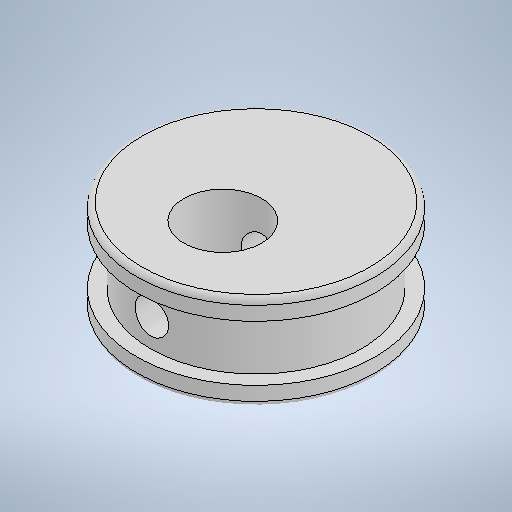
# Autodesk Inventor part: 204
Saved by Autodesk Inventor 2025 (Build 290162010, 162A)
## iProperties
Created: 2024-05-30
Part Number: 204
Material: Generic
Document SubType Name: Modeling
Designer: Fabri
Density: 1 g/cm^3
Appearance: Default
Author: Fabri
Autodesk Inventor part; units mm, degrees
ref_plane "YZ Plane" through (0, 0, 0) normal (1, 0, 0) x (0, 1, 0)
ref_plane "XY Plane" through (0, 0, 0) normal (0, 0, 1) x (1, 0, 0)
sketch "Sketch1" plane through (0, 0, 0) normal (0, 1, 0) x (-1, 0, 0)
  line L0 (0, 0) -> (21.5, 0)
  line L1 (21.5, 0) -> (21.5, -3.5)
  line L2 (21.5, -3.5) -> (19, -3.5)
  line L3 (19, -3.5) -> (19, -13.5)
  line L4 (19, -13.5) -> (21.5, -13.5)
  line L5 (21.5, -13.5) -> (21.5, -17)
  line L6 (21.5, -17) -> (0, -17)
  line L7 (0, -17) -> (0, 0)
  dimension "d1" = 3.5
  dimension "d2" = 3.5
  dimension "d3" = 17
  dimension "d4" = 38
  dimension "d5" = 43
  constraints: 16 end point, 5 perpendicular, 2 point on line, 1 horizontal, 1 vertical
  measures "d1" distance of L0.end L1.end
  measures "d2" distance of L4.end L5.end
  measures "d3" distance between parallel lines of L6 L0
  measures "d4" diameter of L3 L7
  measures "d5" diameter of L5 L7
revolve "Revolution1" add sketch "Sketch1" angle 360 about axis through (0, 0, -17) along (0, 0, 1)
sketch "Sketch2" plane through (0, 0, 0) normal (0, 0, 1) x (1, 0, 0)
  point P0 (0, 0)
  point P1 (0, -6)
  dimension "d14" = 6
  constraints: 1 vertical alignment
  measures "d14" distance of point (0, 0) point (0, -6)
hole "Hole1" at (0, -6, 0) direction (0, 0, -1) diameter 14 depth 17
fillet "Fillet1" radius 1 2 edges at (21.5, 0, 0) (21.5, 0, -17)
ref_plane "Work Plane1" through (0, 20, 0) normal (0, 1, 0) x (-1, 0, 0)
sketch "Sketch4" plane through (0, 20, 0) normal (0, 1, 0) x (-1, 0, 0)
  circle A0 centre (0, -8.5) radius 3
  line L0 (19, -13.5) -> (19, -3.5) projected
  point P0 (0, 0)
  point P1 (19, -8.5)
  dimension "d17" = 6
  constraints: 1 centre point, 1 horizontal alignment, 1 midpoint, 1 vertical alignment
  measures "d17" diameter of A0
extrude "Extrusion1" cut sketch "Sketch4" against normal through all
body "Solid1"
